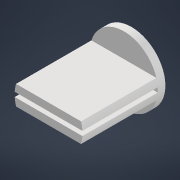
# Autodesk Inventor part: arm - servo mount
Saved by Autodesk Inventor 2021 (Build 250183000, 183)
## iProperties
Created: 2022-05-21
Part Number: arm - servo mount
Material: PET Plastic
Document SubType Name: Modeling
Designer: techv
Mass: 53.2049 g
Surface Area: 164.112 cm^2
Volume: 34.5262 cm^3
Density: 1.541 g/cm^3
Appearance: Polycarbonate - Clear
Author: techv
Autodesk Inventor part; units mm, degrees
ref_plane "YZ Plane" through (0, 0, 0) normal (1, 0, 0) x (0, 1, 0)
ref_plane "XZ Plane" through (0, 0, 0) normal (0, 1, 0) x (-1, 0, 0)
sketch "Sketch1" plane through (0, 0, 0) normal (0, 0, 1) x (1, 0, 0)
  circle A0 centre (0, 0) radius 17.5
  dimension "d0" = 35
  constraints: 1 centre point, 1 coincident
  measures "d0" diameter of A0
extrude "Extrusion1" add sketch "Sketch1" along normal blind 5
sketch "Sketch2" plane through (0, 0, 5) normal (0, 0, 1) x (1, 0, 0)
  line L0 (25, 1.5) -> (-25, 1.5)
  line L1 (-25, 1.5) -> (-25, -1.5)
  line L2 (-25, -1.5) -> (25, -1.5)
  line L3 (25, -1.5) -> (25, 1.5)
  line L4 (25, 1.5) -> (-25, -1.5) construction
  line L5 (-25, 1.5) -> (25, -1.5) construction
  arc A0 (-8.8619, 3.6913) -> (8.9371, 3.5055) centre (0, 0) ccw projected
  circle A1 centre (0, 0) radius 17.5 projected
  circle A2 centre (0, 0) radius 17.5 projected
  line L6 (17.4356, -1.5) -> (-22.5, -1.5)
  line L7 (-22.5, -1.5) -> (-22.5, -6.5)
  line L8 (-22.5, -6.5) -> (17.4356, -6.5)
  line L9 (17.4356, -6.5) -> (17.4356, -1.5)
  line L10 (17.4356, 1.5) -> (-22.5, 1.5)
  line L11 (-22.5, 1.5) -> (-22.5, 6.5)
  line L12 (-22.5, 6.5) -> (17.4356, 6.5)
  line L13 (17.4356, 6.5) -> (17.4356, 1.5)
  point P0 (-3.75, -16.4)
  point P1 (16.2481, 6.5)
  point P2 (-16.2481, 6.5)
  point P3 (-17.4356, 1.5)
  point P4 (17.4356, 1.5)
  point P5 (16.2481, -6.5)
  point P6 (17.4356, -1.5)
  point P7 (-17.4356, -1.5)
  point P8 (-16.2481, -6.5)
  dimension "d3" = 50
  dimension "d4" = 3
  dimension "d5" = 5
  dimension "d6" = 5
  constraints: 28 end point, 6 parallel, 3 horizontal, 3 perpendicular, 3 point on line, 2 midpoint, 2 point on circle, 1 other
  measures "d3" distance of L2.end L1.end
  measures "d4" distance of L1.end L0.end
  measures "d5" distance of L7.end L6.end
  measures "d6" distance of L10.end L11.end
extrude "Extrusion2" add sketch "Sketch2" along normal blind 50 contours L0 A1 L12 | A1 L8 A0 L2 | A0 L8 L2 | A0 L8 A1 L2
sketch "Sketch3" plane through (-16.2481, 6.5, 5) normal (0, 1, 0) x (1, 0, 0)
  line L0 (0, 0) -> (32.4962, 0) projected
  line L1 (0, 0) -> (0, -50) projected
  line L2 (32.4962, -50) -> (0, -50) projected
  line L3 (32.4962, 0) -> (32.4962, -50) projected
  line L4 (0, 0) -> (0, -50) projected
  line L5 (32.4962, 0) -> (32.4962, -50) projected
  line L6 (0, 0) -> (32.4962, -50)
  line L7 (32.4962, -50) -> (0, -50) projected
  line L8 (0, -50) -> (32.4962, 0)
  line L9 (27.6217, -7.5) -> (4.8744, -7.5)
  line L10 (4.8744, -7.5) -> (4.8744, -42.5)
  line L11 (4.8744, -42.5) -> (27.6217, -42.5)
  line L12 (27.6217, -42.5) -> (27.6217, -7.5)
  line L13 (27.6217, -7.5) -> (4.8744, -42.5) construction
  line L14 (4.8744, -7.5) -> (27.6217, -42.5) construction
  circle A0 centre (27.6217, -42.5) radius 1.5
  circle A1 centre (4.8744, -42.5) radius 1.5
  circle A2 centre (4.8744, -7.5) radius 1.5
  circle A3 centre (27.6217, -7.5) radius 1.5
  point P0 (16.2481, 5)
  point P1 (16.2481, -25)
  dimension "d9" = 35
  dimension "d10" = 3
  dimension "d11" = 3
  dimension "d12" = 3
  dimension "d13" = 3
  constraints: 16 end point, 4 centre point, 4 coincident, 3 midpoint, 2 parallel, 1 horizontal, 1 perpendicular, 1 point on line
  measures "d9" distance of L10.end L9.end
  measures "d10" diameter of A0
  measures "d11" diameter of A1
  measures "d12" diameter of A2
  measures "d13" diameter of A3
extrude "Extrusion3" cut sketch "Sketch3" against normal through all contours A2 L9 L6 | L6 L10 A2 | A3 L12 L8 | L8 L9 A3 | A1 L10 L8 | L8 L11 A1 | L9 A2 L6 | L6 A2 L10 | A0 L11 L6 | L6 L12 A0 | L12 A3 L8 | L8 A3 L9 | L10 A1 L8 | L8 A1 L11 | L11 A0 L6 | L6 A0 L12
sketch "Sketch4" plane through (-16.2481, -6.5, 5) normal (0, -1, 0) x (1, 0, 0)
  line L0 (13.75, 50) -> (18.75, 50)
  line L1 (18.75, 50) -> (18.75, 0)
  line L2 (18.75, 0) -> (13.75, 0)
  line L3 (13.75, 0) -> (13.75, 50)
  line L4 (0, 50) -> (32.4962, 50) projected
  line L5 (32.4962, 0) -> (0, 0) projected
  line L6 (0, 0) -> (0, 50) projected
  point P0 (16.2481, -5)
  dimension "d16" = 0
  dimension "d17" = 0
  dimension "d18" = 5
  dimension "d19" = 13.75
  constraints: 8 end point, 2 parallel, 1 horizontal, 1 perpendicular
  measures "d16" distance between parallel lines of L4 L0
  measures "d17" distance between parallel lines of L5 L2
  measures "d18" distance between parallel lines of L1 L3
  measures "d19" distance between parallel lines of L3 L6
ref_plane "Work Plane1" through (-232.5644, -49.9301, 5) normal (0, -1, 0) x (1, 0, 0)
extrude "Extrusion4" add sketch "Sketch4" along normal up to surface (43.4301 mm away) contours L0 L1 L2 L3
sketch "Sketch5" plane through (-2.4981, -6.5, 5) normal (-1, 0, 0) x (0, 0, 1)
  ellipse E0 centre (25.0308, -20) end of major axis (25.0308, -23.5) minor radius 3.5 projected
  point P0 (-5, 6.5)
  constraints: 1 other
extrude "Extrusion5" cut sketch "Sketch5" against normal through all
sketch "Sketch6" plane through (-2.4981, -6.5, 5) normal (-1, 0, 0) x (0, 0, 1)
  circle A0 centre (25.0308, -31.22) radius 2.08 projected
  point P0 (-5, 6.5)
extrude "Extrusion6" cut sketch "Sketch6" against normal up to surface (5 mm away)
sketch "Sketch7" plane through (-2.4981, -6.5, 5) normal (-1, 0, 0) x (0, 0, 1)
  circle A0 centre (33.7808, -40.11) radius 1.5 projected
  circle A1 centre (16.2808, -40.11) radius 1.5 projected
  point P0 (-5, 6.5)
extrude "Extrusion7" cut sketch "Sketch7" against normal blind 50
sketch "Sketch8" plane through (-2.4981, -49.9301, 5) normal (0, -1, 0) x (1, 0, 0)
  line L0 (0, 0) -> (0, 50) projected
  line L1 (5, 0) -> (0, 0) projected
  line L2 (5, 50) -> (5, 0) projected
  line L3 (0, 50) -> (5, 50) projected
  point P0 (2.4981, -5)
extrude "Extrusion8" add sketch "Sketch8" along normal blind 10
body "Solid1"
